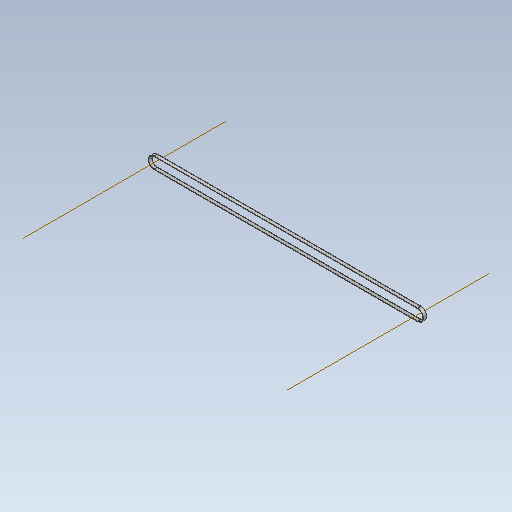
# Autodesk Inventor part: Synchronous Belt
Saved by Autodesk Inventor 2020 (Build 240168000, 168)
## iProperties
Created: 2021-03-06
Part Number: Synchronous Belt
Material: Rubber
Document SubType Name: Modeling
Designer: Harry
Density: 1 g/cm^3
Appearance: Rubber - Black - Version 1.1
CustomPartVersion: 1
Author: Harry
Autodesk Inventor part; units mm, degrees
sketch "Sketch Path" plane through (0, 0, 0) normal (0, 0, 1) x (1, 0, 0)
  arc A0 (0, 8.0851) -> (0, -8.0851) centre (0, 0) ccw
  arc A1 (380, -8.0851) -> (380, 8.0851) centre (380, 0) ccw
  line L0 (380, -8.0851) -> (0, -8.0851)
  line L1 (0, 8.0851) -> (380, 8.0851)
  constraints: 4 end point, 4 point on circle, 2 centre point
ref_plane "Cross Section Plane" through (0, -8.0851, 0) normal (1, 0, 0) x (0, 0, 1)
ref_plane "Work Plane2" through (0, 0, 0) normal (-1, 0, 0) x (0, 0, 1)
ref_plane "Work Plane3" through (380, 0, 0) normal (-0.9691, 0.2468, 0) x (0, 0, 1)
sketch "Cross Section" plane through (0, -8.0851, 0) normal (1, 0, 0) x (0, 0, 1)
  line L0 (-2.413, 0.381) -> (2.413, 0.381)
  line L1 (2.413, 0.381) -> (2.413, -0.254)
  line L2 (2.413, -0.254) -> (-2.413, -0.254)
  line L3 (-2.413, -0.254) -> (-2.413, 0.381)
  line L4 (-2.413, 0) -> (2.413, 0) construction
  point P0 (0, 0)
  point P1 (0, 0)
  dimension "d0" = 4.826
  dimension "d4" = 0.254
  dimension "d5" = 0.381
  constraints: 10 end point, 2 parallel, 2 point on line, 1 coincident, 1 horizontal, 1 midpoint, 1 perpendicular, 1 other
  measures "d0" distance between parallel lines of L1 L3
  measures "d4" distance between parallel lines of L2 L4
  measures "d5" distance between parallel lines of L4 L0
sweep "Belt" add profiles "Cross Section" path "Sketch Path"
equation "\"d0\" = da_B"
equation "\"d4\" = da_a"
equation "\"d5\" = da_a2"
equation "\"da_B\" = 4.826"
equation "\"da_pb\" = 2.032"
equation "\"da_L\" = 810.8"
equation "\"da_a\" = 0.254"
equation "\"da_S\" = 1.143"
equation "\"da_Beta\" = 20deg"
equation "\"da_Ht\" = 0.508"
equation "\"da_H\" = 1.143"
equation "\"da_a2\" = 0.381"
body "Solid1"
